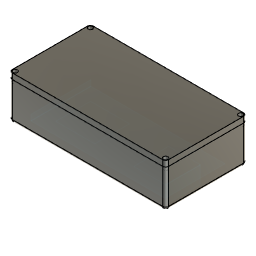
Badminton initial Design v2 (Autodesk Fusion 360 design; units mm, degrees)
Autodesk Fusion 360 part; units mm, degrees
sketch "Sketch1" plane through (0, 0, 0) normal (0, 0, 1) x (1, 0, 0)
  line L0 (-29.4066, 13.5777) -> (20.5934, 13.5777)
  line L1 (20.5934, 13.5777) -> (20.5934, -14.4223)
  line L2 (20.5934, -14.4223) -> (-29.4066, -14.4223)
  line L3 (-29.4066, -14.4223) -> (-29.4066, 13.5777)
  dimension "d1" = 50
  dimension "d2" = 28
  constraint horizontal L0
  constraint vertical L1
  constraint horizontal L2
  constraint vertical L3
  measures "d1" distance of L0.start L0.end
  measures "d2" distance of L0.start L2.end
extrude "Extrude1" add sketch "Sketch1" along normal blind 15 makes body 1
shell "Shell1" thickness 2 outward yes removed faces 0 bodies 1
sketch "Sketch2" plane through (0, -16.4223, 0) normal (0, -1, 0) x (1, 0, 0)
  line L0 (-31.4066, -2) -> (22.5934, -2)
  line L1 (22.5934, -2) -> (22.5934, 17)
  line L2 (22.5934, 17) -> (-31.4066, 17)
  line L3 (-31.4066, 17) -> (-31.4066, -2)
  line L4 (-31.4066, 17) -> (22.5934, 17)
  line L5 (22.5934, 17) -> (22.5934, 14.9315)
  line L6 (22.5934, 14.9315) -> (-31.4066, 14.9315)
  line L7 (-31.4066, 14.9315) -> (-31.4066, 17)
  constraint horizontal L4
  constraint vertical L5
  constraint horizontal L6
  constraint vertical L7
  constraint coincident L1 L5.end
  constraint coincident L2.end L3.start
extrude "Extrude2" cut sketch "Sketch2" against normal blind 67 contours L1 L2 L3 L4 L5 L6 L7 bodies 1
fillet "Fillet1" radius 2 8 edges at (22.5934, -16.4223, 6.4657) (-31.4066, -16.4223, 6.4657) (22.5934, 15.5777, 6.4657) (-31.4066, 15.5777, 6.4657) (-4.4066, 15.5777, -2) (-31.4066, -0.4223, -2) (-4.4066, -16.4223, -2) (22.5934, -0.4223, -2) on bodies 1
sketch "Sketch3" plane through (0, 0, 0) normal (0, 0, 1) x (1, 0, 0)
sketch "Sketch4" plane through (0, 0, 0) normal (0, 0, 1) x (-1, 0, 0)
  line L0 (29.4066, 14.4223) -> (-20.5934, 14.4223)
  line L1 (-20.5934, 14.4223) -> (-20.5934, -13.5777)
  line L2 (-20.5934, -13.5777) -> (29.4066, -13.5777)
  line L3 (29.4066, -13.5777) -> (29.4066, 14.4223)
  line L4 (28, -12) -> (-15.2, -12)
  line L5 (-15.2, -12) -> (-15.2, 5.76)
  line L6 (-15.2, 5.76) -> (28, 5.76)
  line L7 (28, 5.76) -> (28, -12)
  line L8 (28, -12) -> (26.72, -12)
  line L9 (26.72, -12) -> (26.72, 5.76)
  line L10 (26.72, 5.76) -> (28, 5.76)
  line L11 (28, 5.76) -> (28, -12)
  line L12 (-15.2, 5.76) -> (-13.92, 5.76)
  line L13 (-13.92, 5.76) -> (-13.92, -12)
  line L14 (-13.92, -12) -> (-15.2, -12)
  line L15 (-15.2, -12) -> (-15.2, 5.76)
  line L16 (-15.2, 5.76) -> (28, 5.76)
  line L17 (28, 5.76) -> (28, 4.5)
  line L18 (28, 4.5) -> (-15.2, 4.5)
  line L19 (-15.2, 4.5) -> (-15.2, 5.76)
  line L20 (-15.2, -12) -> (28, -12)
  line L21 (28, -12) -> (28, -10.74)
  line L22 (28, -10.74) -> (-15.2, -10.74)
  line L23 (-15.2, -10.74) -> (-15.2, -12)
  circle A0 centre (-13.92, -10.74) radius 0.885
  circle A1 centre (-13.92, 4.5) radius 0.885
  circle A2 centre (26.72, 4.5) radius 0.885
  circle A3 centre (26.72, -10.74) radius 0.885
  dimension "d10" = 43.2
  dimension "d11" = 17.76
  dimension "d12" = 1.28
  dimension "d13" = 1.28
  dimension "d14" = 1.26
  dimension "d15" = 1.26
  dimension "d16" = 1.77
  dimension "d17" = 1.77
  dimension "d18" = 1.77
  dimension "d19" = 1.77
  constraint horizontal L4
  constraint vertical L5
  constraint horizontal L6
  constraint vertical L7
  constraint horizontal L8
  constraint vertical L9
  constraint horizontal L10
  constraint vertical L11
  constraint horizontal L12
  constraint vertical L13
  constraint horizontal L14
  constraint vertical L15
  constraint horizontal L16
  constraint vertical L17
  constraint horizontal L18
  constraint vertical L19
  constraint horizontal L20
  constraint vertical L21
  constraint horizontal L22
  constraint vertical L23
  constraint coincident L22 A0.centre
  constraint coincident L13 A0.centre
  constraint coincident L13 A1.centre
  constraint coincident L18 A1.centre
  constraint coincident L18 A2.centre
  constraint coincident L9 A2.centre
  constraint coincident L9 A3.centre
  constraint coincident L22 A3.centre
  measures "d10" distance of L4.start L4.end
  measures "d11" distance of L4.start L6.end
  measures "d12" distance of L4.start L8.end
  measures "d13" distance of L5.end L12.end
  measures "d14" distance of L5.end L18.end
  measures "d15" distance of L4.end L22.end
  measures "d16" diameter of A0
  measures "d17" diameter of A1
  measures "d18" diameter of A2
  measures "d19" diameter of A3
extrude "Extrude3" add sketch "Sketch4" along normal blind 1 contours L9 L22 A3 | L9 L22 A3 | L9 L22 A3 | L13 L22 A0 | L13 L22 A0 | L9 L22 A3 | L9 L18 A2 | L9 L18 A2 | L13 L22 A0 | L13 L22 A0 | L9 L18 A2 | L9 L18 A2 | L13 L18 A1 | L13 L18 A1 | L13 L18 A1 | L13 L18 A1 bodies 1
sketch "Sketch5" plane through (0, 0, 0) normal (0, 0, 1) x (-1, 0, 0)
  circle A0 centre (26.72, 4.5) radius 0.885
  circle A1 centre (-13.92, 4.5) radius 0.885
  circle A2 centre (26.72, -10.74) radius 0.885
  circle A3 centre (-13.92, -10.74) radius 0.885
  line L0 (29.4066, 14.4223) -> (-20.5934, 14.4223)
  line L1 (-20.5934, 14.4223) -> (-20.5934, -13.5777)
  line L2 (-20.5934, -13.5777) -> (29.4066, -13.5777)
  line L3 (29.4066, -13.5777) -> (29.4066, 14.4223)
  line L4 (29.4066, 7.1886) -> (-16.9976, 7.1886)
  line L5 (-16.9976, 7.1886) -> (-16.9976, -13.5777)
  line L6 (-16.9976, -13.5777) -> (29.4066, -13.5777)
  line L7 (29.4066, -13.5777) -> (29.4066, 7.1886)
  constraint horizontal L4
  constraint vertical L5
  constraint horizontal L6
  constraint vertical L7
  constraint coincident L2 L5.end
  constraint coincident L3 L4.start
extrude "Extrude4" cut sketch "Sketch5" against normal blind 7 contours L0 L1 L2 L3 L4 L5 bodies 1
extrude "Extrude5" cut 1 faces at (-12.74, 14.911, 14.9315) along direction (0, 0, -1) blind 35 on bodies 1 bodies 1
sketch "Sketch6" plane through (0, 0, -2) normal (0, 0, -1) x (1, 0, 0)
  line L0 (16.9976, -13.5777) -> (16.9976, 7.1886)
  line L1 (16.9976, 7.1886) -> (-29.4066, 7.1886)
  line L2 (-29.4066, 7.1886) -> (-29.4066, -13.5777)
  line L3 (-29.4066, -13.5777) -> (16.9976, -13.5777)
  line L4 (13, -9) -> (2, -9)
  line L5 (2, -9) -> (2, 3)
  line L6 (2, 3) -> (13, 3)
  line L7 (13, 3) -> (13, -9)
  line L8 (-25, 3) -> (2, 3)
  line L9 (2, 3) -> (2, -9)
  line L10 (2, -9) -> (-25, -9)
  line L11 (-25, -9) -> (-25, 3)
  line L12 (-11.5, -9) -> (-25, -9)
  line L13 (-25, -9) -> (-25, 3)
  line L14 (-25, 3) -> (-11.5, 3)
  line L15 (-11.5, 3) -> (-11.5, -9)
  constraint horizontal L4
  constraint vertical L5
  constraint horizontal L6
  constraint vertical L7
  constraint horizontal L8
  constraint vertical L9
  constraint horizontal L10
  constraint vertical L11
  constraint horizontal L12
  constraint vertical L13
  constraint horizontal L14
  constraint vertical L15
  constraint midpoint L10 L12.start
extrude "Extrude6" add sketch "Sketch6" along normal blind 6 contours L4 L5 L6 L7 L9 | L8 L10 L11 L12 L13 L14 L15 bodies 1
sketch "Sketch7" plane through (13, 0, 0) normal (1, 0, 0) x (0, 1, 0)
  line L0 (9, -2) -> (-3, -2)
  line L1 (-3, -2) -> (-3, -8)
  line L2 (-3, -8) -> (9, -8)
  line L3 (9, -8) -> (9, -2)
extrude "Extrude7" add 2 faces at (-16, 5, -8) (9.3333, 5, -8) along direction (0, 0, -1) blind 4 on bodies 1 bodies 1
sketch "Sketch8" plane through (-25, 0, 0) normal (-1, 0, 0) x (0, -1, 0)
  line L0 (3, -2) -> (-9, -2)
  line L1 (-9, -2) -> (-9, -12)
  line L2 (-9, -12) -> (3, -12)
  line L3 (3, -12) -> (3, -2)
  circle A0 centre (-3, -7) radius 4.4721
extrude "Extrude8" cut sketch "Sketch8" against normal blind 45 contours A0 bodies 1
sketch "Sketch9" plane through (-25, 0, 0) normal (-1, 0, 0) x (0, -1, 0)
  circle A0 centre (-3, -7) radius 4.4721
  line L0 (3, -2) -> (-9, -2)
  line L1 (-9, -2) -> (-9, -12)
  line L2 (-9, -12) -> (3, -12)
  line L3 (3, -12) -> (3, -2)
  line L4 (3, -8) -> (-9, -8)
  constraint coincident L3 L4.start
  constraint perpendicular L3 L4
extrude "Extrude9" cut sketch "Sketch9" against normal blind 55 contours A0 L1 L2 L3 L4 bodies 1
sketch "Sketch10" plane through (0, 0, -2) normal (0, 0, -1) x (1, 0, 0)
  line L0 (-11.5, 3) -> (-11.5, -9)
  line L1 (-11.5, -9) -> (-25, -9)
  line L2 (-25, -9) -> (-25, 3)
  line L3 (-25, 3) -> (-11.5, 3)
  line L4 (13, 3) -> (13, -9)
  line L5 (13, -9) -> (2, -9)
  line L6 (2, -9) -> (2, 3)
  line L7 (2, 3) -> (13, 3)
  line L8 (16.9976, -13.5777) -> (16.9976, 7.1886)
  line L9 (16.9976, 7.1886) -> (-29.4066, 7.1886)
  line L10 (-29.4066, 7.1886) -> (-29.4066, -13.5777)
  line L11 (-29.4066, -13.5777) -> (16.9976, -13.5777)
sketch "Sketch11" plane through (-29.4066, 0, 0) normal (-1, 0, 0) x (0, -1, 0)
  line L0 (7.1886, 0) -> (-13.5777, 0)
  line L1 (-13.5777, 0) -> (-13.5777, -2)
  line L2 (-13.5777, -2) -> (7.1886, -2)
  line L3 (7.1886, -2) -> (7.1886, 0)
sketch "Sketch12" plane through (0, 0, 0) normal (1, 0, 0) x (0, 1, 0)
sketch "Sketch13" plane through (0, 0, 0) normal (0, 0, 1) x (1, 0, 0)
  line L0 (-31, 15) -> (19, 15)
  line L1 (19, 15) -> (19, -9)
  line L2 (19, -9) -> (-31, -9)
  line L3 (-31, -9) -> (-31, 15)
  constraint horizontal L0
  constraint vertical L1
  constraint horizontal L2
  constraint vertical L3
extrude "Extrude10" add sketch "Sketch13" along normal blind 11 separate body makes body 2
shell "Shell2" thickness 2 outward yes removed faces 0 bodies 2
combine "Combine1" operation add target body 2 tool bodies 1
extrude "Extrude11" cut 1 faces at (-15, 7.6667, 13) along direction (0, 0, -1) blind 1 on bodies 2 bodies 2
extrude "Extrude12" cut 1 faces at (-15, 7.6667, 12) along direction (0, 0, -1) blind 1 on bodies 2 bodies 2
sketch "Sketch14" plane through (0, 0, 11) normal (0, 0, 1) x (-1, 0, 0)
  line L0 (-19, 9) -> (31, 9)
  line L1 (31, 9) -> (31, -15)
  line L2 (31, -15) -> (-19, -15)
  line L3 (-19, -15) -> (-19, 9)
  line L4 (33, 11) -> (-21, 11)
  line L5 (-21, 11) -> (-21, -17)
  line L6 (-21, -17) -> (33, -17)
  line L7 (33, -17) -> (33, 11)
  circle A0 centre (32, 10) radius 0.8
  circle A1 centre (32, -16) radius 0.8
  circle A2 centre (-20, -16) radius 0.8
  circle A3 centre (-20, 10) radius 0.8
  dimension "d41" = 1.6
  dimension "d42" = 1.6
  dimension "d43" = 1.6
  dimension "d44" = 1.6
  measures "d41" diameter of A0
  measures "d42" diameter of A1
  measures "d43" diameter of A2
  measures "d44" diameter of A3
extrude "Extrude13" cut sketch "Sketch14" against normal blind 1 contours A0 | A1 | A2 | A3 bodies 2
fillet "Fillet2" radius 1 8 edges at (-33, 3, -2) (-6, -11, -2) (21, 3, -2) (-6, 17, -2) (21, 17, 4.5) (21, -11, 4.5) (-33, -11, 4.5) (-33, 17, 4.5) on bodies 2
sketch "Sketch15" plane through (-33, 0, 0) normal (-1, 0, 0) x (0, -1, 0)
  line L0 (10, -1) -> (10, 11)
  line L1 (10, 11) -> (-16, 11)
  line L2 (-16, 11) -> (-16, -1)
  line L3 (-16, -1) -> (10, -1)
  line L4 (-10.2729, 4.5474) -> (5.5606, 4.5474)
  line L5 (5.5606, 4.5474) -> (5.5606, 0)
  line L6 (5.5606, 0) -> (-10.2729, 0)
  line L7 (-10.2729, 0) -> (-10.2729, 4.5474)
  constraint horizontal L4
  constraint vertical L5
  constraint horizontal L6
  constraint vertical L7
extrude "Extrude14" cut sketch "Sketch15" against normal blind 3 contours L4 L5 L6 L7 bodies 2
sketch "Sketch16" plane through (-33, 0, 0) normal (-1, 0, 0) x (0, -1, 0)
  line L0 (5.5606, 4.5474) -> (5.5606, 0)
  line L1 (5.5606, 0) -> (-10.2729, 0)
  line L2 (-10.2729, 0) -> (-10.2729, 4.5474)
  line L3 (-10.2729, 4.5474) -> (5.5606, 4.5474)
  line L4 (10, -1) -> (10, 11)
  line L5 (10, 11) -> (-16, 11)
  line L6 (-16, 11) -> (-16, -1)
  line L7 (-16, -1) -> (10, -1)
  line L8 (-10.2729, 4.5474) -> (5.5135, 4.5474)
  line L9 (5.5135, 4.5474) -> (5.5135, 5.9611)
  line L10 (5.5135, 5.9611) -> (-10.2729, 5.9611)
  line L11 (-10.2729, 5.9611) -> (-10.2729, 4.5474)
  constraint horizontal L8
  constraint vertical L9
  constraint horizontal L10
  constraint vertical L11
  constraint coincident L2.end L3.start
extrude "Extrude15" cut sketch "Sketch16" against normal blind 13 contours L3 L8 L9 L10 L11 bodies 2
fillet "Fillet3" radius 2 2 edges at (-32, 10.2729, 5.9611) (-32, -5.5135, 5.9611) on bodies 2
sketch "Sketch17" plane through (0, 0, 0) normal (0, 0, 1) x (1, 0, 0)
  line L0 (-33, 17) -> (21, 17)
  line L1 (21, 17) -> (21, -11)
  line L2 (21, -11) -> (-33, -11)
  line L3 (-33, -11) -> (-33, 17)
  line L4 (-31, 15) -> (19, 15)
  line L5 (19, 15) -> (19, -9)
  line L6 (19, -9) -> (-31, -9)
  line L7 (-31, -9) -> (-31, 15)
  constraint horizontal L0
  constraint vertical L1
  constraint horizontal L2
  constraint vertical L3
  constraint horizontal L4
  constraint vertical L5
  constraint horizontal L6
  constraint vertical L7
extrude "Extrude16" add sketch "Sketch17" along normal blind 2 separate body contours L0 L1 L2 L3 | L4 L5 L6 L7 makes body 3
move_body "Move1" bodies 3 to x (1, 0, 0) y (0, 1, 0) z (0, 0, 1) at (0, 0, 11)
sketch "Sketch18" plane through (0, 0, 0) normal (0, 0, 1) x (1, 0, 0)
sketch "Sketch19" plane through (0, 0, 11) normal (0, 0, 1) x (-1, 0, 0)
  arc A0 (33, 10) -> (32, 11) centre (32, 10) ccw
  line L0 (32, 11) -> (-20, 11)
  arc A1 (-20, 11) -> (-21, 10) centre (-20, 10) ccw
  line L1 (-21, 10) -> (-21, -16)
  arc A2 (-21, -16) -> (-20, -17) centre (-20, -16) ccw
  line L2 (-20, -17) -> (32, -17)
  arc A3 (32, -17) -> (33, -16) centre (32, -16) ccw
  line L3 (33, -16) -> (33, 10)
  circle A4 centre (32, 10) radius 0.8
  circle A5 centre (-20, 10) radius 0.8
  circle A6 centre (32, -16) radius 0.8
  circle A7 centre (-20, -16) radius 0.8
  line L4 (-19, 9) -> (31, 9)
  line L5 (31, 9) -> (31, -15)
  line L6 (31, -15) -> (-19, -15)
  line L7 (-19, -15) -> (-19, 9)
extrude "Extrude17" add sketch "Sketch19" against normal blind 1.5 contours L4 L5 L6 L7 bodies 3
fillet "Fillet4" radius 1 4 edges at (21, -11, 12) (21, 17, 12) (-33, 17, 12) (-33, -11, 12) on bodies 3
sketch "Sketch20" plane through (0, 0, 13) normal (0, 0, 1) x (-1, 0, 0)
  arc A0 (33, 10) -> (32, 11) centre (32, 10) ccw
  line L0 (32, 11) -> (-20, 11)
  arc A1 (-20, 11) -> (-21, 10) centre (-20, 10) ccw
  line L1 (-21, 10) -> (-21, -16)
  arc A2 (-21, -16) -> (-20, -17) centre (-20, -16) ccw
  line L2 (-20, -17) -> (32, -17)
  arc A3 (32, -17) -> (33, -16) centre (32, -16) ccw
  line L3 (33, -16) -> (33, 10)
  circle A4 centre (-20, 10) radius 0.8055
  circle A5 centre (-20, -16) radius 0.781
  circle A6 centre (32, -16) radius 0.7873
  circle A7 centre (32, 10) radius 0.7843
  constraint concentric A1 A4
  constraint concentric A2 A5
  constraint concentric A3 A6
  constraint concentric A0 A7
extrude "Extrude18" cut sketch "Sketch20" against normal blind 2 contours A6 | A7 bodies 3
extrude "Extrude19" cut 1 faces at (19.8337, -10.3657, 10) along direction (0, 0, 1) blind 5 on bodies 2 bodies 3
extrude "Extrude20" cut 1 faces at (19.8337, 15.6343, 10) along direction (0, 0, 1) blind 5 on bodies 2 bodies 3
